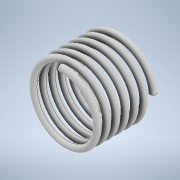
# Autodesk Inventor part: Torsion_Spring_thumb
Saved by Autodesk Inventor 2022 (Build 260153000, 153)
## iProperties
Created: 2023-01-15
Part Number: Torsion_Spring_thumb
Material: Generic
Document SubType Name: Modeling
Designer: 48735
Density: 1 g/cm^3
Appearance: Default
Author: 48735
Autodesk Inventor part; units mm, degrees
ref_plane "YZ Plane" through (0, 0, 0) normal (1, 0, 0) x (0, 1, 0)
ref_plane "XZ Plane" through (0, 0, 0) normal (0, 1, 0) x (-1, 0, 0)
ref_plane "XY Plane" through (0, 0, 0) normal (0, 0, 1) x (1, 0, 0)
sketch "Sketch2" plane through (0, 0, 0) normal (0, 1, 0) x (-1, 0, 0)
  circle A0 centre (-2.75, -1.9689) radius 0.25
  line L0 (0, -1.9689) -> (0, 3.0311)
  point P0 (0, 0)
  dimension "d0" = 0.5
  dimension "d1" = 5
  dimension "d2" = 2.75
  constraints: 2 end point, 1 centre point, 1 vertical
  measures "d0" diameter of A0
  measures "d1" distance of L0.start L0.end
  measures "d2" distance of L0.start A0.centre
coil "Coil1" sketch "Sketch2" operation add axis through (0, 0, -1.9689) along (0, 0, 1) pitch 0.75 turns 6.25 hand right
body "Solid1"
